Autodesk Fusion 360 part; units mm, degrees
(part 3 of 3)
extrude "돌출57" cut sketch "스케치11" against normal blind 4 contours L4 L598 L600 L601 L606 | L4 L663 L665 L666 L671 | L4 L728 L730 L731 L736 | L4 L7 L795 L801 | L7 L794 L797 L799 L800 L802 | L7 L808 L814 L817 | L7 L821 L827 L830 | L7 L807 L810 L812 L813 L815 | L7 L834 L840 L843 | L7 L820 L823 L825 L826 L828 | L6 L7 L853 L856 | L7 L833 L836 L838 L839 L841 | L6 L653 L658 L660 L661 | L6 L718 L723 L725 L726 | L6 L783 L788 L790 L791 | L599 L602 L603 L604 L605 L607 | L611 L613 L614 L619 L621 L622 | L612 L615 L616 L617 L618 L620 | L624 L626 L627 L632 L634 L635 | L625 L628 L629 L630 L631 L633 | L637 L639 L640 L645 L647 L648 | L638 L641 L642 L643 L644 L646 | L664 L667 L668 L669 L670 L672 | L676 L678 L679 L684 L686 L687 | L677 L680 L681 L682 L683 L685 | L689 L691 L692 L697 L699 L700 | L690 L693 L694 L695 L696 L698 | L702 L704 L705 L710 L712 L713 | L703 L706 L707 L708 L709 L711 | L729 L732 L733 L734 L735 L737 | L741 L743 L744 L749 L751 L752 | L742 L745 L746 L747 L748 L750 | L754 L756 L757 L762 L764 L765 | L755 L758 L759 L760 L761 L763 | L767 L769 L770 L775 L777 L778 | L768 L771 L772 L773 L774 L776 bodies 1
extrude "돌출59" cut sketch "스케치11" against normal blind 0.5 contours L4 L5 L26 L29 | L5 L92 L95 L96 L98 L100 | L4 L91 L93 L94 L99 | L5 L39 L42 L49 | L4 L156 L158 L159 L164 | L5 L105 L108 L109 L111 L113 | L4 L221 L223 L224 L229 | L5 L52 L55 L62 | L4 L286 L288 L289 L294 | L5 L118 L121 L122 L124 L126 | L4 L351 L353 L354 L359 | L5 L65 L68 L75 | L4 L416 L418 L419 L424 | L5 L131 L134 L135 L137 L139 | L4 L468 L470 L471 L476 | L5 L6 L81 L88 | L4 L533 L535 L536 L541 | L6 L146 L151 L153 L154 | L6 L211 L216 L218 L219 | L6 L276 L281 L283 L284 | L6 L341 L346 L348 L349 | L6 L406 L411 L413 L414 | L6 L458 L463 L465 L466 | L6 L523 L528 L530 L531 | L6 L588 L593 L595 L596 | L8 L9 L10 L11 L12 L13 | L14 L15 L16 L17 L18 L19 | L104 L106 L107 L112 L114 L115 | L117 L119 L120 L125 L127 L128 | L130 L132 L133 L138 L140 L141 | L157 L160 L161 L162 L163 L165 | L169 L171 L172 L177 L179 L180 | L170 L173 L174 L175 L176 L178 | L182 L184 L185 L190 L192 L193 | L183 L186 L187 L188 L189 L191 | L195 L197 L198 L203 L205 L206 | L196 L199 L200 L201 L202 L204 | L222 L225 L226 L227 L228 L230 | L234 L236 L237 L242 L244 L245 | L235 L238 L239 L240 L241 L243 | L247 L249 L250 L255 L257 L258 | L248 L251 L252 L253 L254 L256 | L260 L262 L263 L268 L270 L271 | L261 L264 L265 L266 L267 L269 | L287 L290 L291 L292 L293 L295 | L299 L301 L302 L307 L309 L310 | L300 L303 L304 L305 L306 L308 | L312 L314 L315 L320 L322 L323 | L313 L316 L317 L318 L319 L321 | L325 L327 L328 L333 L335 L336 | L326 L329 L330 L331 L332 L334 | L352 L355 L356 L357 L358 L360 | L364 L366 L367 L372 L374 L375 | L365 L368 L369 L370 L371 L373 | L377 L379 L380 L385 L387 L388 | L378 L381 L382 L383 L384 L386 | L390 L392 L393 L398 L400 L401 | L391 L394 L395 L396 L397 L399 | L417 L420 L421 L422 L423 L425 | L429 L431 L432 L437 L439 L440 | L430 L433 L434 L435 L436 L438 | L442 L444 L445 L450 L452 L453 | L443 L446 L447 L448 L449 L451 | L469 L472 L473 L474 L475 L477 | L481 L483 L484 L489 L491 L492 | L482 L485 L486 L487 L488 L490 | L494 L496 L497 L502 L504 L505 | L495 L498 L499 L500 L501 L503 | L507 L509 L510 L515 L517 L518 | L508 L511 L512 L513 L514 L516 | L534 L537 L538 L539 L540 L542 | L546 L548 L549 L554 L556 L557 | L547 L550 L551 L552 L553 L555 | L559 L561 L562 L567 L569 L570 | L560 L563 L564 L565 L566 L568 | L572 L574 L575 L580 L582 L583 | L573 L576 L577 L578 L579 L581 bodies 1
fillet "모깎기1" radius 1.5 8 edges at (120.25, 79.3, 66.25) (-37, 79.3, 66.25) (-37, -4, 66.25) (120.25, -4, 66.25) (120.25, 79.3, 134) (-37, 79.3, 134) (-37, -4, 134) (120.25, -4, 134) on bodies 1 2
fillet "모깎기2" radius 3 2 edges at (-31.375, 9.6, 2.5) (-31.375, 75.3, 2.5) on bodies 1
fillet "모깎기3" radius 3 3 edges at (-24, 14.075, 21.5) (-24, 34.475, 21.5) (-24, 54.875, 21.5) on bodies 1
fillet "모깎기4" radius 3 3 edges at (-24, 26.425, 21.5) (-24, 46.825, 21.5) (-24, 67.225, 21.5) on bodies 1
sketch "스케치9" plane through (0, 0, 0) normal (0, 1, 0) x (1, 0, 0)
extrude "돌출42" cut 1 faces at (-31.0833, 9.6, 130.3333) along direction (0, 1, 0) blind 0.3 on bodies 2 bodies 2
extrude "돌출43" cut 3 faces at (-15.5833, 0, 130.8333) (68.4167, 0, 130.8333) (114.9167, 0, 130.8333) along direction (0, 1, 0) blind 0.3 on bodies 2 bodies 2
extrude "돌출44" cut 1 faces at (-34, 53.5, 123.5) along direction (-1, 0, 0) blind 0.3 on bodies 2 bodies 2
extrude "돌출45" cut 1 faces at (116.25, 50.3, 130.8333) along direction (-1, 0, 0) blind 0.3 on bodies 2 bodies 2
extrude "돌출46" cut 1 faces at (-12.25, 1.1, 130.8333) along direction (-1, 0, 0) blind 0.3 on bodies 2 bodies 2
extrude "돌출47" cut 1 faces at (105.25, 1.1, 130.8333) along direction (-1, 0, 0) blind 0.3 on bodies 2 bodies 2
extrude "돌출48" cut 1 faces at (105.25, 74.8, 130.8333) along direction (-1, 0, 0) blind 0.3 on bodies 2 bodies 2
extrude "돌출49" cut 1 faces at (-12.25, 74.8, 130.8333) along direction (-1, 0, 0) blind 0.3 on bodies 2 bodies 2
extrude "돌출50" cut 3 faces at (113.4833, 75.3, 130.8333) (31.4833, 75.3, 130.8333) (-23.9333, 75.3, 130.8333) along direction (0, -1, 0) blind 0.3 on bodies 2 bodies 2
extrude "돌출51" cut 1 faces at (112.25, 74.2, 130.8333) along direction (1, 0, 0) blind 0.3 on bodies 2 bodies 2
extrude "돌출52" cut 1 faces at (-5.25, 74.2, 130.8333) along direction (1, 0, 0) blind 0.3 on bodies 2 bodies 2
extrude "돌출53" cut 1 faces at (-5.25, 0.7, 130.8333) along direction (1, 0, 0) blind 0.3 on bodies 2 bodies 2
extrude "돌출54" cut 1 faces at (112.25, 1.1, 129.1667) along direction (1, 0, 0) blind 0.3 on bodies 2 bodies 2
extrude "돌출55" cut 1 faces at (31.6833, 25.6, 132.5) along direction (0, 0, 1) blind 0.3 on bodies 2 bodies 2
equation "d3 = CARD_HOLES"
equation "d4 = CARD_HOLES"
equation "d5 = CARD_HOLES"
equation "d6 = CARD_HOLES"
equation "CARD_HOLES = 4.35 mm"
equation "d11 = CASE_WALL_OUTER_SIZE"
equation "d12 = CASE_WALL_OUTER_SIZE"
equation "d14 = CASE_WIDTH_FOR_CARD"
equation "d15 = CASE_WALL_OUTER_SIZE"
equation "SLOT_WIDTH = 12.35 mm"
equation "SLOT_GAP = 8.05 mm"
equation "d21 = SLOT_WIDTH"
equation "d24 = SLOT_GAP"
equation "d25 = SLOT_GAP"
equation "d28 = HOLE_GAP"
equation "HOLE_GAP = 0.6 mm"
equation "d33 = HOLE_GAP"
equation "d34 = HOLE_GAP"
equation "CASE_WALL_OUTER_SIZE = 4 mm"
equation "d36 = CONNECTOR_WIDTH"
equation "CONNECTOR_WIDTH = 8.95 mm"
equation "d44 = CONNECTER_GAP"
equation "CONNECTER_GAP = 9.6 mm"
equation "d58 = CASE_BOTTOM_HEIGHT"
equation "d60 = CASE_BOTTOM_HEIGHT"
equation "d62 = MOUNTING_HOLE_HEIGHT"
equation "d64 = CASE_BOTTOM_WALL_HEIGHT"
equation "d66 = SLOT_HEIGHT"
equation "d68 = SLOT_HEIGHT"
equation "d73 = MOUNTING_HOLE_GAP"
equation "d75 = -( CASE_WALL_OUTER_SIZE )"
equation "MOUNTING_HOLE_GAP = MOUNTING_HOLE_HEIGHT + 1.6 mm"
equation "d78 = MOUNTING_HOLE_GAP"
equation "d79 = -( CASE_WALL_OUTER_SIZE )"
equation "SLOT_HEIGHT = CASE_BOTTOM_HEIGHT + 116 mm"
equation "MOUNTING_HOLE_HEIGHT = CASE_BOTTOM_HEIGHT + 9 mm"
equation "SLOT_BOTTOM_HEIGHT = CASE_BOTTOM_HEIGHT + 19 mm"
equation "d90 = SLOT_BOTTOM_HEIGHT"
equation "CASE_BOTTOM_HEIGHT = 2.5 mm"
equation "CASE_BOTTOM_WALL_HEIGHT = CASE_BOTTOM_HEIGHT + 130 mm"
equation "d98 = CASE_BOTTOM_HEIGHT + 4 mm"
equation "d114 = CASE_BOTTOM_WALL_HEIGHT"
equation "d142 = -( CASE_BOTTOM_WALL_HEIGHT - SLOT_HEIGHT - 7.5 mm )"
equation "d152 = CASE_BOTTOM_WALL_HEIGHT"
equation "d157 = CASE_BOTTOM_WALL_HEIGHT"
equation "d190 = CASE_CHAR_SIZE_FOR_CARD"
equation "d191 = CASE_CHAR_SIZE_FOR_CARD + ( CASE_CHAR_SIZE_FOR_CARD / 8 )"
equation "d193 = CASE_CHAR_SIZE_FOR_CARD + ( CASE_CHAR_SIZE_FOR_CARD / 2 )"
equation "d194 = CASE_CHAR_SIZE_FOR_CARD + ( CASE_CHAR_SIZE_FOR_CARD / 2 )"
equation "d216 = -( CASE_BOTTOM_WALL_HEIGHT - SLOT_HEIGHT )"
equation "Tolerance = 0.3 mm"
equation "d252 = -Tolerance"
equation "d254 = -Tolerance"
equation "d256 = -Tolerance"
equation "d258 = -Tolerance"
equation "d260 = -Tolerance"
equation "d262 = -Tolerance"
equation "d264 = -Tolerance"
equation "d266 = -Tolerance"
equation "d268 = -Tolerance"
equation "d270 = -Tolerance"
equation "d272 = -Tolerance"
equation "d274 = -Tolerance"
equation "d276 = -Tolerance"
equation "d278 = -Tolerance"
equation "d282 = MOUNTING_HOLE_HEIGHT + 20 mm"
equation "d302 = -( CASE_WALL_OUTER_SIZE )"
equation "CASE_WIDTH_FOR_CARD = 30 mm"
equation "CASE_CHAR_SIZE_FOR_CARD = 9 mm"
named bodies: "Base", "Top"
